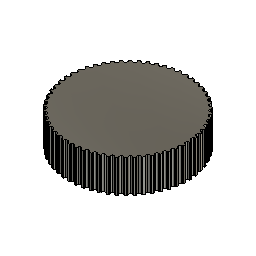
gear_58z (Autodesk Fusion 360 design; units mm, degrees)
Autodesk Fusion 360 part; units mm, degrees
sketch "Sketch1" plane through (0, 0, 0) normal (0, 0, 1) x (1, 0, 0) in component "gt2 pulley"
  circle A0 centre (0, 0) radius 18.462 construction
  circle A1 centre (0, 0) radius 17.458 construction
  line L0 (0, 0) -> (0, 18.462) construction
  line L1 (0, 0) -> (0.9995, 18.4349) construction
  line L2 (0, 0) -> (1.4064, 18.4083) construction
  circle A2 centre (0, 0) radius 18.208 construction
  arc A3 (0.3908, 18.0692) -> (0.4615, 17.7764) centre (1.3871, 18.1551) ccw
  circle A4 centre (0, 0) radius 18.058 construction
  arc A5 (0.2432, 18.2063) -> (0, 18.208) centre (0, 0) ccw
  arc A6 (0.3908, 18.0692) -> (0.2432, 18.2063) centre (0.2413, 18.0564) ccw
  arc A7 (0.4615, 17.7764) -> (0.9452, 17.4324) centre (0.9752, 17.9866) ccw
  arc A8 (0, 18.208) -> (-0.2432, 18.2063) centre (0, 0) ccw
  arc A9 (-0.2432, 18.2063) -> (-0.3908, 18.0692) centre (-0.2413, 18.0564) ccw
  arc A10 (-0.4615, 17.7764) -> (-0.3908, 18.0692) centre (-1.3871, 18.1551) ccw
  arc A11 (-0.945, 17.4324) -> (-0.4615, 17.7764) centre (-0.9752, 17.9865) ccw
  arc A12 (0.9452, 17.4324) -> (-0.9452, 17.4324) centre (0, 0) ccw
  point P0 (1.3871, 18.1551)
  point P1 (0, 18.208)
  dimension "d18" = 36.9239
  dimension "d19" = 3.103
  dimension "d22" = 1.004
  dimension "d24" = 0.75
  dimension "d26" = 1
  dimension "d27" = 0.15
  dimension "d28" = 0.15
  dimension "d47" = 0.555
  dimension "d52" = 3.812
  constraint coincident A0.centre A1.centre
  constraint coincident A0 L0.end
  constraint vertical L0
  constraint coincident A0 L1.end
  constraint coincident A0 L2.end
  constraint concentric A1 A2
  constraint coincident A1 A7.end
  constraint coincident L1 A7.end
  constraint coincident A2 P0
  constraint coincident L2 P0
  constraint coincident P0 A3.centre
  constraint coincident A2 P1
  constraint coincident L0 P1
  constraint concentric A2 A4
  constraint coincident P1 A5.end
  constraint coincident A4 A6.centre
  constraint coincident A3.start A6.start
  constraint tangent A3 A6
  constraint tangent A3 A7
  constraint symmetric L0 A7.end A12.end
  constraint symmetric L0 A3.start A9.end
  constraint symmetric L0 A3.end A10.start
  constraint symmetric L0 A3 A10
  constraint symmetric L0 A5.start A8.end
  constraint symmetric L0 P1 A5.end
  constraint symmetric L0 A5 A8
  constraint symmetric L0 A6 A9
  constraint symmetric L0 A7 A11
  constraint coincident A1 A11.start
  constraint tangent A1 A7
  constraint coincident L1 A7.centre
  measures "d18" diameter of A0
  measures "d19" angle of L0 L1
  measures "d22" distance of A0 A1
  measures "d24" distance of A1 A2
  measures "d26" radius of A3
  measures "d27" distance of A2 A4
  measures "d28" radius of A6
  measures "d47" radius of A7
extrude "Extrude1" add sketch "Sketch1" along normal blind 10 makes body 1
pattern_circular "C-Pattern1" count 58 over 360 about axis through (0, 0, 1.75) along (0, 0, 1) of bodies 1 makes body 2 at (-2.6167, 17.2608, 6.6667) makes body 3 at (-4.4676, 16.8767, 6.6667) makes body 4 at (-5.6737, 16.5103, 6.6667) makes body 5 at (-7.9911, 15.5217, 6.6667) makes body 6 at (-9.0903, 14.9046, 6.6667) makes body 7 at (-9.9704, 14.3308, 3.3333) makes body 8 at (-12.5289, 12.1576, 6.6667) makes body 9 at (-13.7699, 10.7317, 6.6667) makes body 10 at (-14.8495, 9.18, 6.6667) makes body 11 at (-15.755, 7.5207, 6.6667) makes body 12 at (-16.4758, 5.7732, 6.6667) makes body 13 at (-16.8494, 4.5693, 6.6667) makes body 14 at (-17.2447, 2.7207, 6.6667) makes body 15 at (-17.4377, 0.8403, 6.6667) makes body 16 at (-17.3771, -1.6784, 6.6667) makes body 17 at (-17.2107, -2.9279, 6.6667) makes body 18 at (-16.61, -5.3747, 6.6667) makes body 19 at (-16.4758, -5.7731, 3.3333) makes body 20 at (-15.3749, -8.2701, 6.6667) makes body 21 at (-14.3906, -9.8839, 6.6667) makes body 22 at (-13.77, -10.7316, 3.3333) makes body 23 at (-11.4615, -13.1687, 6.6667) makes body 24 at (-10.4814, -13.9615, 6.6667) makes body 25 at (-8.9104, -15.0128, 6.6667) makes body 26 at (-6.6567, -16.139, 6.6667) makes body 27 at (-4.8728, -16.7642, 6.6667) makes body 28 at (-3.6504, -17.0721, 6.6667) makes body 29 at (-1.7831, -17.3667, 6.6667) makes body 30 at (0.7351, -17.4425, 6.6667) makes body 31 at (2.6167, -17.2608, 6.6667) makes body 32 at (3.8554, -17.0269, 6.6667) makes body 33 at (5.6737, -16.5103, 6.6667) makes body 34 at (6.6566, -16.1391, 3.3333) makes body 35 at (9.0903, -14.9046, 6.6667) makes body 36 at (11.141, -13.441, 6.6667) makes body 37 at (12.5289, -12.1576, 6.6667) makes body 38 at (13.7699, -10.7317, 6.6667) makes body 39 at (14.8495, -9.18, 6.6667) makes body 40 at (15.4732, -8.0846, 6.6667) makes body 41 at (16.4758, -5.7732, 6.6667) makes body 42 at (16.8494, -4.5693, 6.6667) makes body 43 at (17.2447, -2.7207, 6.6667) makes body 44 at (17.4567, -0.2103, 6.6667) makes body 45 at (17.3771, 1.6784, 6.6667) makes body 46 at (17.0938, 3.5473, 6.6667) makes body 47 at (17.0034, 3.9579, 3.3333) makes body 48 at (16.4758, 5.7731, 3.3333) makes body 49 at (15.3749, 8.2701, 6.6667) makes body 50 at (14.3906, 9.8839, 6.6667) makes body 51 at (12.8181, 11.8523, 6.6667) makes body 52 at (11.4615, 13.1687, 6.6667) makes body 53 at (9.9705, 14.3307, 6.6667) makes body 54 at (9.6226, 14.5666, 3.3333) makes body 55 at (6.6567, 16.139, 6.6667) makes body 56 at (4.8728, 16.7642, 6.6667) makes body 57 at (3.6504, 17.0721, 6.6667) makes body 58 at (1.7831, 17.3667, 6.6667)
sketch "Sketch2" plane through (0, 0, 10) normal (0, 0, 1) x (-1, 0, 0)
  arc A0 (-14.0247, -11.4) -> (-14.0337, -11.6011) centre (-13.9181, -11.5055) ccw
  arc A1 (-14.0337, -11.6011) -> (-13.7187, -11.9719) centre (0, 0) ccw
  arc A2 (-13.7187, -11.9719) -> (-13.5187, -11.9956) centre (-13.6057, -11.8734) ccw
  arc A3 (-13.2497, -11.86) -> (-13.5187, -11.9956) centre (-12.9391, -12.8105) ccw
  arc A4 (-12.6745, -12.0057) -> (-13.2497, -11.86) centre (-13.0773, -12.3875) ccw
  arc A5 (-13.8982, -10.5651) -> (-12.6745, -12.0057) centre (0, 0) ccw
  arc A6 (-13.8473, -11.1564) -> (-13.8982, -10.5651) centre (-14.34, -10.901) ccw
  arc A7 (-14.0247, -11.4) -> (-13.8473, -11.1564) centre (-14.7351, -10.6962) ccw
  circle A8 centre (0, 0) radius 17.458
  constraint coincident A1.centre A5.centre
extrude "Extrude2" add sketch "Sketch2" against normal blind 10 contours A5 A8 bodies 1 2 3 4 5 6 7 8 9 10 11 12 13 14 15 16 17 18 19 20 21 22 23 24 25 26 27 28 29 30 31 32 33 34 35 36 37 38 39 40 41 42 43 44 45 46 47 48 49 50 51 52 53 54 55 56 57 58
extrude "Extrude4" [suppressed] in component "gt2 pulley"
pattern_circular "C-Pattern7" [suppressed] in component "gt2 pulley"
extrude "Extrude3" [suppressed] in component "gt2 pulley"
pattern_circular "C-Pattern6" [suppressed] in component "gt2 pulley"
extrude "Extrude2'" [suppressed] in component "gt2 pulley"
pattern_circular "C-Pattern5" [suppressed] in component "gt2 pulley"
extrude "Extrude1'" [suppressed] in component "gt2 pulley"
pattern_circular "C-Pattern4" [suppressed] in component "gt2 pulley"
pattern_circular "C-Pattern3" [suppressed] in component "gt2 pulley"
pattern_circular "C-Pattern2" [suppressed] in component "gt2 pulley"
pattern_circular "C-Pattern1'" [suppressed] in component "gt2 pulley"
copy_body "Body->Comp1" [suppressed] in component "Component"
copy_body "Body->Comp2" [suppressed] in component "Component'"
copy_body "Body->Comp3" [suppressed] in component "Component''"
copy_body "Body->Comp4" [suppressed] in component "Component'''"
copy_body "Body->Comp5" [suppressed] in component "Component''''"
copy_body "Body->Comp6" [suppressed] in component "Component'''''"
copy_body "Body->Comp7" [suppressed] in component "Component''''''"
copy_body "Body->Comp8" [suppressed] in component "Component'''''''"
copy_body "Body->Comp9" [suppressed] in component "Component''''''''"
copy_body "Body->Comp10" [suppressed] in component "Component'''''''''"
copy_body "Body->Comp11" [suppressed] in component "Component''''''''''"
copy_body "Body->Comp12" [suppressed] in component "Component'''''''''''"
copy_body "Body->Comp13" [suppressed] in component "Component''''''''''''"
copy_body "Body->Comp14" [suppressed] in component "Component'''''''''''''"
copy_body "Body->Comp15" [suppressed] in component "Component''''''''''''''"
copy_body "Body->Comp16" [suppressed] in component "Component'''''''''''''''"
copy_body "Body->Comp17" [suppressed] in component "Component''''''''''''''''"
copy_body "Body->Comp18" [suppressed] in component "Component'''''''''''''''''"
copy_body "Body->Comp19" [suppressed] in component "Component''''''''''''''''''"
copy_body "Body->Comp20" [suppressed] in component "Component'''''''''''''''''''"
component "gt2 pulley" placed x (1, 0, 0) y (0, 1, 0) z (0, 0, 1) at (0, 0, 0)
equation "NumTeeth = 58" comment "min 20"
equation "ToothPitch = 2 mm"
equation "PullyDia = NumTeeth * ToothPitch / PI"
equation "ToothAng = ( ( 360 / NumTeeth ) * 1 deg )"
equation "TransOffsetAngle = ToothAng * 0.2"
equation "Sholulder_Radius = 0.15 mm"
equation "Root_Radius = 0.555 mm"
equation "TransRadius = 1 mm"
equation "ToolHeight = 0.75 mm"
equation "PLD = 0.254 mm"
equation "d18 = PullyDia"
equation "d19 = ToothAng / 2"
equation "d22 = PLD + ToolHeight"
equation "d24 = ToolHeight"
equation "d26 = TransRadius"
equation "d27 = Sholulder_Radius"
equation "d31 = NumTeeth"
equation "d33 = NumTeeth"
equation "d35 = NumTeeth"
equation "d37 = NumTeeth"
equation "d41 = NumTeeth"
equation "d45 = NumTeeth"
equation "d47 = Root_Radius"
equation "d50 = NumTeeth"
